# Autodesk Inventor part: ADR3425ARJZ-R7
Saved by Autodesk Inventor 2016 (Build 200138000, 138)
## iProperties
Created: 2016-04-08
Part Number: ADR3425ARJZ-R7
Material: Generic
Document SubType Name: Modeling
Designer: Paschalis
Density: 1 g/cm^3
Appearance: SOT95P280X145-6N, ADR3425ARJZ-R7
Author: Paschalis
Autodesk Inventor part; units mm, degrees
ref_plane "YZ Plane" through (0, 0, 0) normal (1, 0, 0) x (0, 1, 0)
ref_plane "XZ Plane" through (0, 0, 0) normal (0, 1, 0) x (-1, 0, 0)
ref_plane "XY Plane" through (0, 0, 0) normal (0, 0, 1) x (1, 0, 0)
sketch "SOT95P280X145-6N, ADR3425ARJZ-R7_3" plane through (0, 0, 0) normal (0, 0, 1) x (1, 0, 0)
  line L0 (-1.4986, 1.4986) -> (1.4986, 1.4986)
  line L1 (1.4986, 1.4986) -> (1.4986, -1.5748)
  line L2 (1.4986, -1.5748) -> (-1.4986, -1.5748)
  line L3 (-1.4986, -1.5748) -> (-1.4986, 1.4986)
  constraints: 8 end point
extrude "Extrusion1" add sketch "SOT95P280X145-6N, ADR3425ARJZ-R7_3" along normal blind 1
body "Solid1"
